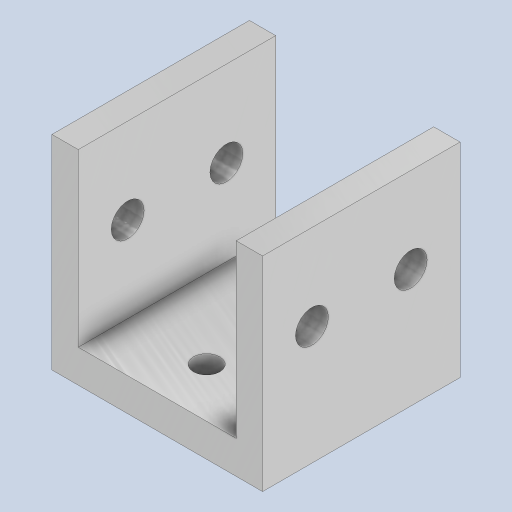
# Autodesk Inventor part: Suporte da célula de carga
Saved by Autodesk Inventor 2023 (Build 270158000, 158)
## iProperties
Created: 2023-03-25
Part Number: Suporte da célula de carga
Material: Aço galvanizado
Document SubType Name: Sheet Metal
Designer: Mateus
Density: 7.85 g/cm^3
Sheet Metal Rule: Default_mm
Appearance: Usinado - Alumínio
Mass: 88.7745 g
Surface Area: 69.1531 cm^2
Volume: 11.3088 cm^3
Author: Mateus
Autodesk Inventor part; units mm, degrees
ref_plane "YZ Plane" through (0, 0, 0) normal (1, 0, 0) x (0, 1, 0)
ref_plane "XZ Plane" through (0, 0, 0) normal (0, 1, 0) x (-1, 0, 0)
ref_plane "XY Plane" through (0, 0, 0) normal (0, 0, 1) x (1, 0, 0)
sketch "Esboço1" plane through (0, 0, 0) normal (0, 1, 0) x (-1, 0, 0)
  line L0 (0, 0) -> (32, 0)
  line L1 (32, 0) -> (32, -30)
  line L2 (32, -30) -> (0, -30)
  line L3 (0, -30) -> (0, 0)
  dimension "d0" = 32
  dimension "d1" = 30
  constraints: 8 end point, 2 parallel, 1 horizontal, 1 perpendicular
  measures "d0" distance of L1.end L2.end
  measures "d1" distance of L0.end L1.end
extrude "Extrusion1" add sketch "Esboço1" along normal blind 5
sketch "Sketch4" plane through (0, 5, 0) normal (0, 1, 0) x (1, 0, 0)
  line L0 (-32, 30) -> (-28, 30)
  line L1 (-28, 30) -> (-28, 0)
  line L2 (-28, 0) -> (-32, 0)
  line L3 (-32, 0) -> (-32, 30)
  line L4 (-4, 30) -> (0, 30)
  line L5 (0, 30) -> (0, 0)
  line L6 (0, 0) -> (-4, 0)
  line L7 (-4, 0) -> (-4, 30)
  dimension "d59" = 24
  constraints: 16 end point, 4 parallel, 2 equal length, 2 horizontal, 2 perpendicular
  measures "d59" distance of L0.end L4.start
extrude "Extrusion2" add sketch "Sketch4" along normal blind 26
sketch "Sketch5" plane through (0, 0, 0) normal (1, 0, 0) x (0, 0, -1)
  line L0 (0, 0) -> (0, 31) projected
  line L1 (30, 0) -> (30, 31) projected
  line L2 (0, 31) -> (30, 31) projected
  point P0 (7.5, 18)
  point P1 (22.5, 18)
  dimension "d30" = 7.5
  dimension "d31" = 7.5
  dimension "d32" = 13
  dimension "d33" = 13
  measures "d30" distance from line of L0 point (7.5, 18)
  measures "d31" distance from line of L1 point (22.5, 18)
  measures "d32" distance from line of L2 point (22.5, 18)
  measures "d33" distance from line of L2 point (7.5, 18)
hole "Hole2" at (0, 18, -7.5) at (0, 18, -22.5) direction (-1, 0, 0) diameter 5 end through all
sketch "Esboço6" plane through (0, 5, 0) normal (0, 1, 0) x (1, 0, 0)
  line L0 (-4, 30) -> (-28, 30) projected
  line L1 (-28, 0) -> (-28, 30) projected
  line L2 (-32, 30) -> (-32, 0) projected
  line L3 (-4, 30) -> (-4, 0) projected
  point P0 (0, 0)
  point P1 (-16, 22.5)
  point P2 (-16, 7.5)
  dimension "d43" = 15
  dimension "d45" = 24
  dimension "d48" = 30
  dimension "d57" = 12
  dimension "d58" = 7.5
  constraints: 1 vertical alignment
  measures "d43" distance of point (-16, 22.5) point (-16, 7.5)
  measures "d45" distance of L0.start L0.end
  measures "d48" distance of L1.start L0.end
  measures "d57" distance from line of L3 point (-16, 22.5)
  measures "d58" distance from line of L0 point (-16, 22.5)
hole "Furo3" at (-16, 5, -22.5) at (-16, 5, -7.5) direction (0, -1, 0) diameter 4 depth 5
equation "\"d31\" = d30"
equation "\"d33\" = d32"
equation "\"d39\" = Espessura"
equation "\"d57\" = 0.5 * d45"
equation "\"d58\" = -0.5 * d43 + 0.5 * d48"
equation "\"d55\" = Espessura"
equation "\"Raio_vergadura\" = Espessura"
equation "\"Largura_alívio_de_vergadura\" = Espessura"
equation "\"Profundidade_alívio_de_vergadura\" = 0.5 * Espessura"
equation "\"Raiodetransição\" = Raio_vergadura"
equation "\"Tamanho_de_raio_de_Jacobi\" = Raio_vergadura"
equation "\"TamanhoFolga\" = Espessura"
equation "\"Espessura\" = 5"
body "Solid2"
